battery upper holder (Autodesk Fusion 360 design; units mm, degrees)
Autodesk Fusion 360 part; units mm, degrees
sketch "Sketch1" plane through (0, 0, 0) normal (0, 1, 0) x (1, 0, 0)
  circle A0 centre (0, 0) radius 3
  circle A1 centre (0, 0) radius 5
  line L0 (0, 0) -> (-50, 0) construction
  circle A2 centre (-50, 0) radius 3
  circle A3 centre (-50, 0) radius 5
  line L1 (-50, -5) -> (0, -5)
  line L2 (0, 5) -> (-50, 5)
  dimension "d1" = 6
  dimension "d2" = 10
  dimension "d3" = 50
  dimension "d4" = 6
  dimension "d5" = 10
  constraint coincident A0.centre A1.centre
  constraint horizontal L0
  constraint coincident L0.end A2.centre
  constraint concentric A2 A3
  constraint coincident A3 L1.start
  constraint coincident A1 L1.end
  constraint tangent A1 L1
  constraint coincident A1 L2.start
  constraint coincident A3 L2.end
  constraint tangent A3 L2
  constraint tangent A3 L1
  constraint tangent A1 L2
  measures "d1" diameter of A0
  measures "d2" diameter of A1
  measures "d3" distance of A0.centre L0.end
  measures "d4" diameter of A2
  measures "d5" diameter of A3
extrude "Extrude1" add sketch "Sketch1" along normal blind 10
sketch "Sketch2" plane through (0, 10, 0) normal (0, 1, 0) x (-1, 0, 0)
  circle A0 centre (50, 0) radius 3
  circle A1 centre (0, 0) radius 3
  line L0 (0, -5) -> (50, -5)
  arc A2 (50, -5) -> (50, 5) centre (50, 0) ccw
  line L1 (50, 5) -> (0, 5)
  arc A3 (0, 5) -> (0, -5) centre (0, 0) ccw
  line L2 (11, 5) -> (39, 5)
  line L3 (39, 5) -> (39, -5)
  line L4 (39, -5) -> (11, -5)
  line L5 (11, -5) -> (11, 5)
  dimension "d8" = 28
  constraint horizontal L2
  constraint vertical L3
  constraint horizontal L4
  constraint vertical L5
  constraint midpoint L1 L2
  constraint coincident L0 L3.end
  measures "d8" distance of L3.end L4.end
extrude "Extrude2" add sketch "Sketch2" along normal blind 40 contours L0 L1 L2 L3 L4 L5
sketch "Sketch3" plane through (0, 0, 5) normal (0, 0, 1) x (-1, 0, 0)
  line L0 (50, 0) -> (0, 0)
  line L1 (0, 0) -> (0, -10)
  line L2 (0, -10) -> (11, -10)
  line L3 (11, -10) -> (11, -50)
  line L4 (11, -50) -> (39, -50)
  line L5 (39, -50) -> (39, -10)
  line L6 (39, -10) -> (50, -10)
  line L7 (50, -10) -> (50, 0)
  line L8 (11, -10) -> (39, -10) construction
  line L9 (25, -10) -> (25, -15) construction
  line L10 (34, -45.5) -> (16, -45.5)
  line L11 (16, -45.5) -> (16, -15)
  line L12 (16, -15) -> (34, -15)
  line L13 (34, -15) -> (34, -45.5)
  dimension "d11" = 5
  dimension "d12" = 18
  dimension "d13" = 30.5
  constraint coincident L2.end L3.start
  constraint coincident L5.end L6.start
  constraint midpoint L8 L9.start
  constraint perpendicular L8 L9
  constraint horizontal L10
  constraint vertical L11
  constraint horizontal L12
  constraint vertical L13
  constraint midpoint L9.end L12
  measures "d11" distance of L9.start L9.end
  measures "d12" distance of L11.end L12.end
  measures "d13" distance of L10.end L11.end
extrude "Extrude3" cut sketch "Sketch3" against normal blind 10 contours L10 L11 L12 L13
